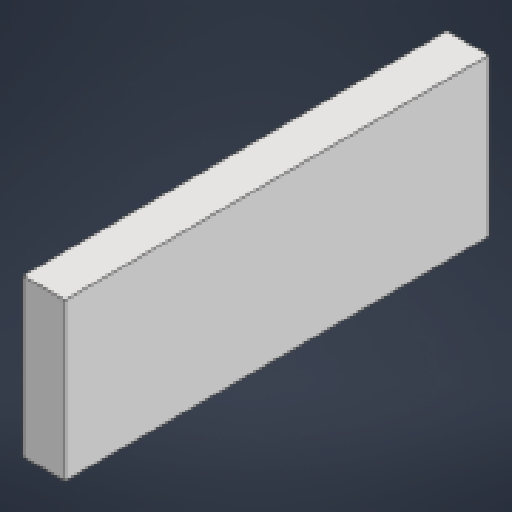
# Autodesk Inventor part: nut
Saved by Autodesk Inventor 2024 (Build 280153000, 153)
## iProperties
Created: 2024-05-04
Part Number: nut
Material: Steel, Alloy
Document SubType Name: Modeling
Designer: markm
Density: 7.73 g/cm^3
Appearance: Semi-Polished
Author: markm
Autodesk Inventor part; units mm, degrees
ref_plane "YZ Plane" through (0, 0, 0) normal (1, 0, 0) x (0, 1, 0)
ref_plane "XZ Plane" through (0, 0, 0) normal (0, 1, 0) x (-1, 0, 0)
ref_plane "XY Plane" through (0, 0, 0) normal (0, 0, 1) x (1, 0, 0)
sketch "Sketch14" plane through (0, 0, 0) normal (0, 0, 1) x (1, 0, 0)
  line L0 (0, 0) -> (26.230089, 0)
  line L1 (0, -13.5) -> (0, -6.375)
  line L2 (0, -6.375) -> (13, -6.375)
  line L3 (13, -6.375) -> (13, -9.5)
  line L4 (10.5, -12) -> (4, -12)
  line L5 (4, -12) -> (4, -13.5)
  line L6 (4, -13.5) -> (0, -13.5)
  arc A0 (10.5, -12) -> (13, -9.5) centre (10.5, -9.5) ccw
  point P0 (13, -12)
  dimension "d94" = 27
  dimension "d95" = 12.75
  dimension "d96" = 24
  dimension "d97" = 4
  dimension "d98" = 13
  dimension "d108" = 2.5
  constraints: 14 end point, 5 perpendicular, 3 point on line, 2 point on circle, 2 tangent, 1 centre point, 1 horizontal, 1 vertical
  measures "d94" diameter of L6 L0
  measures "d95" diameter of L2 L0
  measures "d96" diameter of L4 L0
  measures "d97" distance of L5.end L1.start
  measures "d98" distance of L1.end L2.end
  measures "d108" radius of A0
sketch "Sketch14 outline for Revolution1" plane through (0, 0, 0) normal (0, 0, 1) x (1, 0, 0)
  line L0 (4, -12) -> (10.5, -12)
  line L1 (4, -13.5) -> (4, -12)
  line L2 (0, -13.5) -> (4, -13.5)
  line L3 (0, -6.375) -> (0, -13.5)
  line L4 (13, -6.375) -> (0, -6.375)
  line L5 (13, -9.5) -> (13, -6.375)
  arc A0 (10.5, -12) -> (13, -9.5) centre (10.5, -9.5) ccw
revolve "Revolution1" add sketch "Sketch14 outline for Revolution1" angle 360 about axis through (0, 0, 0) along (1, 0, 0)
sketch "Sketch15" plane through (13, 0, 0) normal (1, 0, 0) x (0, 0, -1)
  line L0 (-6, -10.392305) -> (-12, 0)
  line L1 (-12, 0) -> (-6, 10.392305)
  line L2 (-6, 10.392305) -> (6, 10.392305)
  line L3 (6, 10.392305) -> (12, 0)
  line L4 (12, 0) -> (6, -10.392305)
  line L5 (6, -10.392305) -> (-6, -10.392305)
  circle A0 centre (0, 0) radius 12
  constraints: 12 end point, 1 coincident, 1 horizontal, 1 point on circle, 13 other
sketch "Sketch15 outline for Extrusion11" plane through (13, 0, 0) normal (1, 0, 0) x (0, 0, -1)
  arc A0 (6, -10.392305) -> (12, 0) centre (0, 0) ccw
  line L0 (12, 0) -> (6, -10.392305)
  arc A1 (12, 0) -> (6, 10.392305) centre (0, 0) ccw
  line L1 (6, 10.392305) -> (12, 0)
  arc A2 (6, 10.392305) -> (-6, 10.392305) centre (0, 0) ccw
  line L2 (-6, 10.392305) -> (6, 10.392305)
  arc A3 (-6, 10.392305) -> (-12, 0) centre (0, 0) ccw
  line L3 (-12, 0) -> (-6, 10.392305)
  arc A4 (-12, 0) -> (-6, -10.392305) centre (0, 0) ccw
  line L4 (-6, -10.392305) -> (-12, 0)
  arc A5 (-6, -10.392305) -> (6, -10.392305) centre (0, 0) ccw
  line L5 (6, -10.392305) -> (-6, -10.392305)
extrude "Extrusion11" cut sketch "Sketch15 outline for Extrusion11" against normal blind 9 contours L0 A0 | A5 L5 | L1 A1 | A4 L4 | L2 A2 | A3 L3
thread "Thread1" size "M14x2" class "6H" standard "ANSI Metric M Profile" full length
chamfer "Chamfer2" distance 3 distance2 1.5 1 edges at (4, 13.5, 0)
fillet "Fillet8" radius 1 2 edges at (0, 13.5, 0) (2.5, 13.5, 0)
chamfer "Chamfer3" distance 1 angle 45 2 edges at (0, 6.375, 0) (13, 6.375, 0)
body "Solid4"
